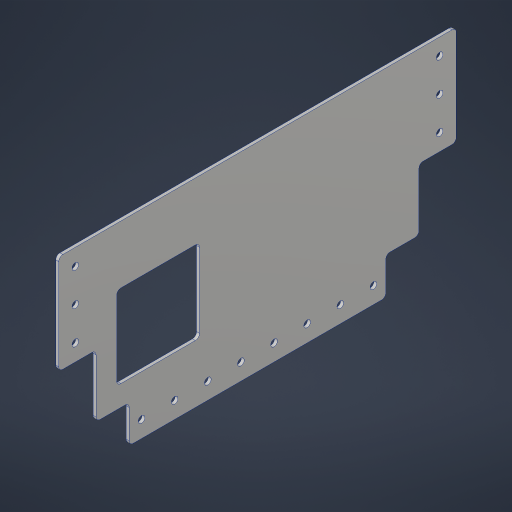
# Autodesk Inventor part: DB1-025
Saved by Autodesk Inventor 2023.4 (Build 274418000, 418)
## iProperties
Created: 2025-03-10
Part Number: DB1-025
Material: Aluminum 6061
Document SubType Name: Modeling
Designer: brand
Density: 2.7 g/cm^3
Appearance: Aluminum - Flat
Author: brand
Autodesk Inventor part; units mm, degrees
ref_plane "YZ Plane" through (0, 0, 0) normal (1, 0, 0) x (0, 1, 0)
ref_plane "XZ Plane" through (0, 0, 0) normal (0, 1, 0) x (-1, 0, 0)
ref_plane "XY Plane" through (0, 0, 0) normal (0, 0, 1) x (1, 0, 0)
sketch "Sketch1" plane through (0, 0, 0) normal (1, 0, 0) x (0, 1, 0)
  line L0 (76.2, 152.4) -> (-76.2, 152.4)
  line L1 (-76.2, 152.4) -> (-76.2, -152.4)
  line L2 (-76.2, -152.4) -> (76.2, -152.4)
  line L3 (76.2, -152.4) -> (76.2, 152.4)
  line L4 (76.2, 152.4) -> (-76.2, -152.4) construction
  line L5 (-76.2, 152.4) -> (76.2, -152.4) construction
  line L6 (31.75, 107.95) -> (-31.75, 107.95)
  line L7 (-31.75, 107.95) -> (-31.75, 44.45)
  line L8 (-31.75, 44.45) -> (31.75, 44.45)
  line L9 (31.75, 44.45) -> (31.75, 107.95)
  line L10 (31.75, 107.95) -> (-31.75, 44.45) construction
  line L11 (-31.75, 107.95) -> (31.75, 44.45) construction
  point P0 (0, 0)
  point P1 (0, 76.2)
  dimension "d0" = 152.4
  dimension "d1" = 304.8
  dimension "d2" = 63.5
  dimension "d3" = 76.2
  dimension "d4" = 76.2
  constraints: 24 end point, 4 midpoint, 4 parallel, 3 perpendicular, 2 horizontal
  measures "d0" distance of L2.end L1.end
  measures "d1" distance of L1.end L0.end
  measures "d2" distance of L8.end L6.start
  measures "d3" distance from line of L1 point (0, 76.2)
  measures "d4" distance from line of point (0, 76.2) L0
extrude "Extrusion1" add sketch "Sketch1" along normal blind 2.286
fillet "Fillet1" radius 3.175 8 edges at (1.143, 31.75, 44.45) (1.143, 31.75, 107.95) (1.143, -31.75, 107.95) (1.143, -31.75, 44.45) (1.143, 76.2, 152.4) (1.143, 76.2, -152.4) (1.143, -76.2, -152.4) (1.143, -76.2, 152.4)
sketch "Sketch2" plane through (2.286, 0, 0) normal (1, 0, 0) x (0, 0, -1)
  arc A0 (-152.4, -73.025) -> (-149.225, -76.2) centre (-149.225, -73.025) ccw construction
  line L0 (-152.4, -73.025) -> (-152.4, 73.025) construction
  arc A1 (-149.225, 76.2) -> (-152.4, 73.025) centre (-149.225, 73.025) ccw construction
  line L1 (-149.225, 76.2) -> (149.225, 76.2) construction
  arc A2 (152.4, 73.025) -> (149.225, 76.2) centre (149.225, 73.025) ccw construction
  line L2 (152.4, 73.025) -> (152.4, -73.025) construction
  arc A3 (149.225, -76.2) -> (152.4, -73.025) centre (149.225, -73.025) ccw construction
  line L3 (149.225, -76.2) -> (-149.225, -76.2) construction
  arc A4 (-47.625, -31.75) -> (-44.45, -28.575) centre (-47.625, -28.575) ccw construction
  line L4 (-44.45, -28.575) -> (-44.45, 28.575) construction
  arc A5 (-44.45, 28.575) -> (-47.625, 31.75) centre (-47.625, 28.575) ccw construction
  line L5 (-47.625, 31.75) -> (-104.775, 31.75) construction
  arc A6 (-104.775, 31.75) -> (-107.95, 28.575) centre (-104.775, 28.575) ccw construction
  line L6 (-107.95, 28.575) -> (-107.95, -28.575) construction
  arc A7 (-107.95, -28.575) -> (-104.775, -31.75) centre (-104.775, -28.575) ccw construction
  line L7 (-104.775, -31.75) -> (-47.625, -31.75) construction
  point P0 (0, 0)
  point P1 (-139.7, -63.5)
  point P2 (139.7, -63.5)
  point P3 (-139.7, -38.1)
  point P4 (139.7, -38.1)
  point P5 (-139.7, -12.7)
  point P6 (139.7, -12.7)
  point P7 (-139.7, 12.7)
  point P8 (139.7, 12.7)
  point P9 (-139.7, 38.1)
  point P10 (139.7, 38.1)
  point P11 (-139.7, 63.5)
  point P12 (139.7, 63.5)
  point P13 (-114.3, -63.5)
  point P14 (-88.9, -63.5)
  point P15 (-63.5, -63.5)
  point P16 (-38.1, -63.5)
  point P17 (-12.7, -63.5)
  point P18 (12.7, -63.5)
  point P19 (38.1, -63.5)
  point P20 (63.5, -63.5)
  point P21 (88.9, -63.5)
  point P22 (114.3, -63.5)
  point P23 (139.7, -63.5)
  dimension "d8" = 12.7
  dimension "d9" = 12.7
  dimension "d10" = 12.7
  dimension "d13" = 25.4
  dimension "d34" = 25.4
  constraints: 1 horizontal, 1 horizontal alignment, 1 vertical, 21 other
  measures "d8" distance from line of L0 point (-139.7, -63.5)
  measures "d9" distance from line of L2 point (139.7, -63.5)
  measures "d10" distance from line of L3 point (139.7, -63.5)
  measures "d13" distance of point (-139.7, -63.5) point (-139.7, -38.1)
  measures "d34" distance of point (-139.7, -63.5) point (-114.3, -63.5)
hole "Hole1" at (2.286, -63.5, 139.7) at (2.286, -63.5, -139.7) at (2.286, -38.1, 139.7) at (2.286, -38.1, -139.7) at (2.286, -12.7, 139.7) at (2.286, -12.7, -139.7) at (2.286, 12.7, 139.7) at (2.286, 12.7, -139.7) at (2.286, 38.1, 139.7) at (2.286, 38.1, -139.7) at (2.286, 63.5, 139.7) at (2.286, 63.5, -139.7) at (2.286, -63.5, 88.9) at (2.286, -63.5, 63.5) at (2.286, -63.5, 38.1) at (2.286, -63.5, 12.7) at (2.286, -63.5, -12.7) at (2.286, -63.5, -38.1) at (2.286, -63.5, -63.5) at (2.286, -63.5, -88.9) direction (-1, 0, 0) diameter 5.1054 end through all clearance for "Flat Head Machine Screw (82)" size "#10" standard "Ansi Unified Screw Threads"
sketch "Sketch3" plane through (2.286, 0, 0) normal (1, 0, 0) x (0, 0, -1)
  line L0 (-123.825, 0) -> (-152.4, 0)
  line L1 (-152.4, 0) -> (-152.4, -76.2)
  line L2 (-152.4, -76.2) -> (-123.825, -76.2)
  line L3 (-123.825, -76.2) -> (-123.825, 0)
  line L4 (-123.825, 0) -> (-152.4, -76.2) construction
  line L5 (-152.4, 0) -> (-123.825, -76.2) construction
  circle A0 centre (-139.7, 63.5) radius 2.5527 construction
  circle A1 centre (-139.7, 38.1) radius 2.5527 construction
  circle A2 centre (-139.7, 12.7) radius 2.5527 construction
  circle A3 centre (-139.7, -12.7) radius 2.5527 construction
  circle A4 centre (-139.7, -38.1) radius 2.5527 construction
  circle A5 centre (-139.7, -63.5) radius 2.5527 construction
  circle A6 centre (139.7, -63.5) radius 2.5527 construction
  circle A7 centre (139.7, -38.1) radius 2.5527 construction
  circle A8 centre (139.7, -12.7) radius 2.5527 construction
  circle A9 centre (139.7, 12.7) radius 2.5527 construction
  circle A10 centre (139.7, 38.1) radius 2.5527 construction
  circle A11 centre (139.7, 63.5) radius 2.5527 construction
  arc A12 (-152.4, -73.025) -> (-149.225, -76.2) centre (-149.225, -73.025) ccw construction
  line L6 (-152.4, -73.025) -> (-152.4, 73.025) construction
  arc A13 (-149.225, 76.2) -> (-152.4, 73.025) centre (-149.225, 73.025) ccw construction
  line L7 (-149.225, 76.2) -> (149.225, 76.2) construction
  arc A14 (152.4, 73.025) -> (149.225, 76.2) centre (149.225, 73.025) ccw construction
  line L8 (152.4, 73.025) -> (152.4, -73.025) construction
  arc A15 (149.225, -76.2) -> (152.4, -73.025) centre (149.225, -73.025) ccw construction
  line L9 (149.225, -76.2) -> (-149.225, -76.2) construction
  arc A16 (-47.625, -31.75) -> (-44.45, -28.575) centre (-47.625, -28.575) ccw construction
  line L10 (-44.45, -28.575) -> (-44.45, 28.575) construction
  arc A17 (-44.45, 28.575) -> (-47.625, 31.75) centre (-47.625, 28.575) ccw construction
  line L11 (-47.625, 31.75) -> (-104.775, 31.75) construction
  arc A18 (-104.775, 31.75) -> (-107.95, 28.575) centre (-104.775, 28.575) ccw construction
  line L12 (-107.95, 28.575) -> (-107.95, -28.575) construction
  arc A19 (-107.95, -28.575) -> (-104.775, -31.75) centre (-104.775, -28.575) ccw construction
  line L13 (-104.775, -31.75) -> (-47.625, -31.75) construction
  line L14 (-149.225, -76.2) -> (149.225, -76.2) construction
  line L15 (149.225, 76.2) -> (-149.225, 76.2) construction
  line L16 (0, 76.2) -> (0, -76.2) construction
  line L17 (-149.225, -76.2) -> (149.225, -76.2) construction
  line L18 (-152.4, -47.625) -> (-98.425, -47.625)
  line L19 (-98.425, -47.625) -> (-98.425, -76.2)
  line L20 (-98.425, -76.2) -> (-152.4, -76.2)
  line L21 (-152.4, -76.2) -> (-152.4, -47.625)
  line L22 (-152.4, -47.625) -> (-98.425, -76.2) construction
  line L23 (-98.425, -47.625) -> (-152.4, -76.2) construction
  line L24 (123.825, 0) -> (152.4, 0)
  line L25 (152.4, 0) -> (152.4, -76.2)
  line L26 (152.4, -76.2) -> (123.825, -76.2)
  line L27 (123.825, -76.2) -> (123.825, 0)
  line L28 (123.825, 0) -> (152.4, -76.2) construction
  line L29 (152.4, 0) -> (123.825, -76.2) construction
  circle A20 centre (139.7, -12.7) radius 2.5527 construction
  circle A21 centre (139.7, -38.1) radius 2.5527 construction
  circle A22 centre (139.7, -63.5) radius 2.5527 construction
  arc A23 (149.225, -76.2) -> (152.4, -73.025) centre (149.225, -73.025) ccw construction
  arc A24 (104.775, -31.75) -> (107.95, -28.575) centre (104.775, -28.575) ccw construction
  line L30 (152.4, -47.625) -> (98.425, -47.625)
  line L31 (98.425, -47.625) -> (98.425, -76.2)
  line L32 (98.425, -76.2) -> (152.4, -76.2)
  line L33 (152.4, -76.2) -> (152.4, -47.625)
  line L34 (152.4, -47.625) -> (98.425, -76.2) construction
  line L35 (98.425, -47.625) -> (152.4, -76.2) construction
  circle A25 centre (63.5, -63.5) radius 2.5527 projected
  circle A26 centre (12.7, -63.5) radius 2.5527 projected
  circle A27 centre (-38.1, -63.5) radius 2.5527 projected
  circle A28 centre (-88.9, -63.5) radius 2.5527 projected
  circle A29 centre (-63.5, -63.5) radius 2.5527 projected
  circle A30 centre (-12.7, -63.5) radius 2.5527 projected
  circle A31 centre (38.1, -63.5) radius 2.5527 projected
  circle A32 centre (88.9, -63.5) radius 2.5527 projected
  point P0 (0, 0)
  point P1 (-138.1125, -38.1)
  point P2 (-125.4125, -61.9125)
  point P3 (138.1125, -38.1)
  point P4 (125.4125, -61.9125)
  point P5 (123.825, -47.625)
  point P6 (-123.825, -47.625)
  dimension "d25" = 28.575
  dimension "d26" = 76.2
  dimension "d27" = 28.575
  dimension "d28" = 53.975
  constraints: 50 end point, 17 symmetric about line, 6 midpoint, 5 centre point, 4 collinear, 4 parallel, 4 point on circle, 2 horizontal, 2 perpendicular, 5 other
  measures "d25" distance of L0.start L0.end
  measures "d26" distance of L0.end L1.end
  measures "d27" distance of L20.end L18.start
  measures "d28" distance of L19.end L20.end
extrude "Extrusion2" cut sketch "Sketch3" against normal blind 2.286 contours L3 L18 L1 L0 | L18 L19 L20 L3 | L3 L2 L1 L18 | L24 L25 L30 L27 | L30 L25 L26 L27 | L27 L32 L31 L30
fillet "Fillet2" radius 3.175 10 edges at (1.143, 0, 152.4) (1.143, 0, 123.825) (1.143, -47.625, 123.825) (1.143, -47.625, 98.425) (1.143, -76.2, 98.425) (1.143, -76.2, -98.425) (1.143, -47.625, -98.425) (1.143, -47.625, -123.825) (1.143, 0, -123.825) (1.143, 0, -152.4)
equation "\"d9\" = d8"
equation "\"d10\" = d8"
body "Solid1"
